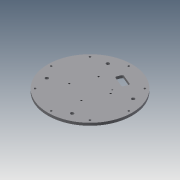
# Autodesk Inventor part: CPU면 철판가공
Saved by Autodesk Inventor 2018 (Build 220112000, 112)
## iProperties
Created: 2018-10-26
Part Number: CPU면 철판가공
Material: 일반
Document SubType Name: Modeling
Designer: dhksr
Density: 1 g/cm^3
Appearance: 기본값
Author: dhksr
Autodesk Inventor part; units mm, degrees
ref_plane "YZ Plane" through (0, 0, 0) normal (1, 0, 0) x (0, 1, 0)
ref_plane "XZ Plane" through (0, 0, 0) normal (0, 1, 0) x (-1, 0, 0)
ref_plane "XY Plane" through (0, 0, 0) normal (0, 0, 1) x (1, 0, 0)
sketch "스케치1" plane through (0, 0, 0) normal (0, 0, 1) x (1, 0, 0)
  line L0 (-18, -16) -> (-18, 16)
  line L1 (-18, 16) -> (18, 16)
  line L2 (18, 16) -> (18, -16)
  line L3 (18, -16) -> (-18, -16)
  circle A0 centre (36.125, 36.075) radius 2.5
  circle A1 centre (-36.125, -36.075) radius 2.5
  circle A2 centre (36.075, -36.125) radius 2.5
  circle A3 centre (-36.075, 36.125) radius 2.5
  arc A4 (-39.6581, -32.537) -> (-32.5919, -39.613) centre (-36.125, -36.075) ccw
  line L4 (-32.5919, -39.613) -> (-17.9206, -24.962)
  arc A5 (-14.3876, -23.5) -> (-17.9206, -24.962) centre (-14.3876, -28.5) ccw
  line L5 (-14.3876, -23.5) -> (14.3282, -23.5)
  arc A6 (17.8662, -24.9669) -> (14.3282, -23.5) centre (14.3282, -28.5) ccw
  line L6 (17.8662, -24.9669) -> (32.537, -39.6581)
  arc A7 (32.537, -39.6581) -> (39.613, -32.5919) centre (36.075, -36.125) ccw
  line L7 (39.613, -32.5919) -> (24.962, -17.9206)
  arc A8 (23.5, -14.3876) -> (24.962, -17.9206) centre (28.5, -14.3876) ccw
  line L8 (23.5, -14.3876) -> (23.5, 14.3282)
  arc A9 (24.9669, 17.8662) -> (23.5, 14.3282) centre (28.5, 14.3282) ccw
  line L9 (24.9669, 17.8662) -> (39.6581, 32.537)
  arc A10 (39.6581, 32.537) -> (32.5919, 39.613) centre (36.125, 36.075) ccw
  line L10 (32.5919, 39.613) -> (17.9206, 24.962)
  arc A11 (14.3876, 23.5) -> (17.9206, 24.962) centre (14.3876, 28.5) ccw
  line L11 (14.3876, 23.5) -> (-14.3282, 23.5)
  arc A12 (-17.8662, 24.9669) -> (-14.3282, 23.5) centre (-14.3282, 28.5) ccw
  line L12 (-17.8662, 24.9669) -> (-32.537, 39.6581)
  arc A13 (-32.537, 39.6581) -> (-39.613, 32.5919) centre (-36.075, 36.125) ccw
  line L13 (-39.613, 32.5919) -> (-24.962, 17.9206)
  arc A14 (-23.5, 14.3876) -> (-24.962, 17.9206) centre (-28.5, 14.3876) ccw
  line L14 (-23.5, 14.3876) -> (-23.5, -14.3282)
  arc A15 (-24.9669, -17.8662) -> (-23.5, -14.3282) centre (-28.5, -14.3282) ccw
  line L15 (-24.9669, -17.8662) -> (-39.6581, -32.537)
  circle A16 centre (0, 0) radius 65
  dimension "d38" = 72.2
  dimension "d39" = 72.2
  dimension "d62" = 130
  constraints: 32 end point, 24 point on circle, 17 centre point, 1 coincident
  measures "d38" distance of A2.centre A4.centre
  measures "d39" distance of A0.centre A2.centre
  measures "d62" diameter of A16
extrude "돌출3" add sketch "스케치1" along normal blind 4 contours L0 L1 L2 L3 | A0 | A1 | A2 | A3 | L15 A15 L14 A14 L13 A13 L12 A12 L11 A11 L10 A10 L9 A9 L8 A8 L7 A7 L6 A6 L5 A5 L4 A4 | A16
sketch "스케치6" plane through (0, 0, 4) normal (0, 0, 1) x (1, 0, 0)
  line L0 (0, 0) -> (60.0652, -60.0652) construction
  line L1 (0, 0) -> (84.945, 0) construction
  circle A0 centre (42.4264, -42.4264) radius 1.5
  circle A1 centre (0, 0) radius 60 construction
  circle A2 centre (0, 0) radius 60 construction
  circle A3 centre (60, 0) radius 1.5
  circle A4 centre (0, 0) radius 60 construction
  circle A5 centre (42.4264, 42.4264) radius 1.5
  circle A6 centre (0, 0) radius 60 construction
  circle A7 centre (0, 60) radius 1.5
  circle A8 centre (0, 0) radius 60 construction
  circle A9 centre (-42.4264, 42.4264) radius 1.5
  circle A10 centre (0, 0) radius 60 construction
  circle A11 centre (-60, 0) radius 1.5
  circle A12 centre (0, 0) radius 60 construction
  circle A13 centre (-42.4264, -42.4264) radius 1.5
  circle A14 centre (0, 0) radius 60 construction
  circle A15 centre (0, -60) radius 1.5
  circle A16 centre (0, 0) radius 65 projected
  dimension "d65" = 120
  dimension "d63" = 45
  dimension "d64" = 3
  dimension "d68" = 360
  dimension "d72" = 130
  constraints: 8 centre point, 4 end point, 2 horizontal alignment, 2 vertical alignment, 1 coincident, 1 equal length, 1 horizontal, 1 point on line, 53 other
  measures "d63" angle of L0 L1
  measures "d64" diameter of A0
  measures "d72" diameter of A16
extrude "돌출4" cut sketch "스케치6" against normal through all contours A0 | A3 | A5 | A7 | A9 | A11 | A13 | A15
sketch "스케치7" plane through (0, 0, 4) normal (0, 0, 1) x (1, 0, 0)
  circle A0 centre (-36.075, 36.125) radius 2.5 projected
  circle A1 centre (36.075, -36.125) radius 2.5 projected
  circle A2 centre (-36.125, -36.075) radius 2.5 projected
  circle A3 centre (36.125, 36.075) radius 2.5 projected
  circle A4 centre (-42.4264, -42.4264) radius 1.5 projected
  circle A5 centre (-42.4264, 42.4264) radius 1.5 projected
  circle A6 centre (42.4264, 42.4264) radius 1.5 projected
  circle A7 centre (42.4264, -42.4264) radius 1.5 projected
  circle A8 centre (60, 0) radius 1.5 projected
  circle A9 centre (0, 60) radius 1.5 projected
  circle A10 centre (-60, 0) radius 1.5 projected
  circle A11 centre (0, -60) radius 1.5 projected
  circle A12 centre (-42.4264, -42.4264) radius 1.5 projected
  circle A13 centre (-42.4264, 42.4264) radius 1.5 projected
  circle A14 centre (42.4264, 42.4264) radius 1.5 projected
  circle A15 centre (42.4264, -42.4264) radius 1.5 projected
  circle A16 centre (60, 0) radius 1.5 projected
  circle A17 centre (0, 60) radius 1.5 projected
  circle A18 centre (-60, 0) radius 1.5 projected
  circle A19 centre (0, -60) radius 1.5 projected
  circle A20 centre (0, 0) radius 65 projected
  circle A21 centre (-36.075, 36.125) radius 2.5
  circle A22 centre (36.125, 36.075) radius 2.5
  circle A23 centre (-36.125, -36.075) radius 2.5
  circle A24 centre (36.075, -36.125) radius 2.5
  circle A25 centre (-47.1805, -19.5045) radius 2.5
  circle A26 centre (19.5045, -47.1805) radius 2.5
  circle A27 centre (47.1805, 19.5045) radius 2.5
  circle A28 centre (-19.5045, 47.1805) radius 2.5
  dimension "d76" = 67.5
  constraints: 16 centre point, 4 coincident, 4 concentric, 9 other
extrude "돌출5" cut sketch "스케치7" against normal through all contours A25 | A26 | A27 | A28
sketch "스케치8" plane through (0, 0, 4) normal (0, 0, 1) x (1, 0, 0)
  circle A0 centre (-19.5045, 47.1805) radius 2.5 projected
  circle A1 centre (0, 0) radius 65 projected
  circle A2 centre (0, 0) radius 24.5 construction
  line L0 (0, 0) -> (-19.5045, 47.1805) construction
  point P0 (-9.3601, 22.6415)
  dimension "d80" = 49
  constraints: 2 end point, 1 coincident, 1 point on line, 3 other
hole "구멍5" at (-9.3601, 22.6415, 4) direction (0, 0, -1) diameter 2.459 end through all thread size "M3x0.5" class "6H" standard "ISO Metric profile"
pattern_circular "원형 패턴1" count 4 over 360 about axis through (0, 0, 0) along (0, 0, 1) of "구멍5"
sketch "스케치9" plane through (0, 0, 0) normal (0, 0, -1) x (-1, 0, 0)
  circle A0 centre (42.4264, 42.4264) radius 1.5 projected
  circle A1 centre (0, 60) radius 1.5 projected
  circle A2 centre (-42.4264, 42.4264) radius 1.5 projected
  circle A3 centre (-60, 0) radius 1.5 projected
  circle A4 centre (-42.4264, -42.4264) radius 1.5 projected
  circle A5 centre (0, -60) radius 1.5 projected
  circle A6 centre (42.4264, -42.4264) radius 1.5 projected
  circle A7 centre (60, 0) radius 1.5 projected
  circle A8 centre (18.5456, 40.1536) radius 1.5 projected
  circle A9 centre (-41.5066, 15.2792) radius 1.5 projected
  circle A10 centre (41.5066, -15.2792) radius 1.5 projected
  circle A11 centre (-18.5456, -40.1536) radius 1.5 projected
  circle A12 centre (0, 0) radius 65 projected
  line L0 (-4.3465, 36.6246) -> (-6.6426, 42.1678) projected
  line L1 (-9.2557, 43.2502) -> (-24.0378, 37.1273) projected
  line L2 (-25.1202, 34.5142) -> (-22.8241, 28.9709) projected
  arc A13 (-37.7646, 20.6175) -> (-38.847, 18.0044) centre (-36.9993, 18.7698) ccw projected
  line L3 (-38.847, 18.0044) -> (-37.699, 15.2327) projected
  arc A14 (-38.7814, 12.6196) -> (-37.699, 15.2327) centre (-39.5467, 14.4674) ccw projected
  line L4 (-38.7814, 12.6196) -> (-41.553, 11.4716) projected
  arc A15 (-41.553, 11.4716) -> (-42.6354, 8.8584) centre (-40.7876, 9.6238) ccw projected
  line L5 (-42.6354, 8.8584) -> (-23.8839, -36.4117) projected
  arc A16 (-23.8839, -36.4117) -> (-21.2708, -37.494) centre (-22.0362, -35.6463) ccw projected
  line L6 (-21.2708, -37.494) -> (-18.4992, -36.346) projected
  arc A17 (-15.886, -37.4284) -> (-18.4992, -36.346) centre (-17.7338, -38.1938) ccw projected
  line L7 (-15.886, -37.4284) -> (-14.738, -40.2) projected
  arc A18 (-14.738, -40.2) -> (-12.1249, -41.2824) centre (-12.8902, -39.4347) ccw projected
  line L8 (-12.1249, -41.2824) -> (37.7646, -20.6175) projected
  arc A19 (37.7646, -20.6175) -> (38.847, -18.0044) centre (36.9993, -18.7698) ccw projected
  line L9 (38.847, -18.0044) -> (37.699, -15.2327) projected
  arc A20 (38.7814, -12.6196) -> (37.699, -15.2327) centre (39.5467, -14.4674) ccw projected
  line L10 (38.7814, -12.6196) -> (41.553, -11.4716) projected
  arc A21 (41.553, -11.4716) -> (42.6354, -8.8584) centre (40.7876, -9.6238) ccw projected
  line L11 (42.6354, -8.8584) -> (23.8839, 36.4117) projected
  arc A22 (23.8839, 36.4117) -> (21.2708, 37.494) centre (22.0362, 35.6463) ccw projected
  line L12 (21.2708, 37.494) -> (18.4992, 36.346) projected
  arc A23 (15.886, 37.4284) -> (18.4992, 36.346) centre (17.7338, 38.1938) ccw projected
  line L13 (15.886, 37.4284) -> (14.738, 40.2) projected
  arc A24 (14.738, 40.2) -> (12.1249, 41.2824) centre (12.8902, 39.4347) ccw projected
  line L14 (12.1249, 41.2824) -> (-1.7333, 35.5422) projected
  line L15 (-7.4079, 44.0156) -> (-25.8789, 36.346)
  line L16 (-25.8789, 36.346) -> (-22.0507, 27.1264)
  line L17 (-7.4079, 44.0156) -> (-3.5797, 34.796)
  line L18 (-3.5797, 34.796) -> (-22.0507, 27.1264)
  constraints: 8 end point, 2 perpendicular
extrude "돌출6" cut sketch "스케치9" against normal through all contours L17 L18 L16 L15
fillet "모깎기1" radius 2 4 edges at (25.8789, 36.346, 2) (22.0507, 27.1264, 2) (3.5797, 34.796, 2) (7.4079, 44.0156, 2)
sketch "스케치10" plane through (0, 0, 4) normal (0, 0, 1) x (1, 0, 0)
  line L0 (25.112, 34.4989) -> (22.8177, 28.9735) projected
  arc A0 (20.2036, 27.8934) -> (22.8177, 28.9735) centre (20.9706, 29.7405) ccw projected
  line L1 (20.2036, 27.8934) -> (5.4268, 34.0291) projected
  arc A1 (4.3467, 36.6431) -> (5.4268, 34.0291) centre (6.1938, 35.8762) ccw projected
  line L2 (4.3467, 36.6431) -> (6.641, 42.1685) projected
  arc A2 (9.255, 43.2486) -> (6.641, 42.1685) centre (8.4881, 41.4015) ccw projected
  line L3 (9.255, 43.2486) -> (24.0318, 37.113) projected
  arc A3 (25.112, 34.4989) -> (24.0318, 37.113) centre (23.2649, 35.2659) ccw projected
  circle A4 centre (22.6415, 9.3601) radius 1.2295 projected
  circle A5 centre (9.3601, -22.6415) radius 1.2295 projected
  circle A6 centre (-22.6415, -9.3601) radius 1.2295 projected
  circle A7 centre (-9.3601, 22.6415) radius 1.2295 projected
  circle A8 centre (47.1805, 19.5045) radius 2.5 projected
  circle A9 centre (-47.1805, -19.5045) radius 2.5 projected
  circle A10 centre (19.5045, -47.1805) radius 2.5 projected
  circle A11 centre (-19.5045, 47.1805) radius 2.5 projected
  circle A12 centre (-42.4264, -42.4264) radius 1.5 projected
  circle A13 centre (-42.4264, 42.4264) radius 1.5 projected
  circle A14 centre (42.4264, 42.4264) radius 1.5 projected
  circle A15 centre (42.4264, -42.4264) radius 1.5 projected
  circle A16 centre (60, 0) radius 1.5 projected
  circle A17 centre (0, 60) radius 1.5 projected
  circle A18 centre (-60, 0) radius 1.5 projected
  circle A19 centre (0, -60) radius 1.5 projected
  circle A20 centre (0, 0) radius 65 projected
  circle A21 centre (0, 0) radius 29 projected
  line L4 (0, 0) -> (59.5002, 0) construction
  circle A22 centre (18.9196, 15.5659) radius 1
  line L5 (18.9196, 15.5659) -> (0, 0)
  circle A23 centre (0, 0) radius 24.5 construction
  dimension "d96" = 2
  constraints: 4 end point, 2 centre point, 2 point on circle, 1 coincident, 1 horizontal
  measures "d96" diameter of A22
extrude "돌출7" cut sketch "스케치10" against normal through all contours A22
